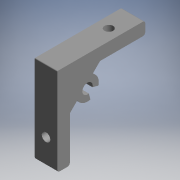
# Autodesk Inventor part: HBLTBS3
Saved by Autodesk Inventor 2017.3 (Build 213256000, 256)
## iProperties
Part Number: HBLTBS3
Material: Generic
Catalog Web Link: www.cadenas.de
Description: HBLTBS3-Square Nuts for Aluminum Extrusions 15mm Square - Extruded Brackets
Vendor: MISUMI
Document SubType Name: Modeling
Designer: partserver
Manufacturer: MISUMI
Mass: 3.67944 g
Surface Area: 22.5843 cm^2
Volume: 3.67944 cm^3
Density: 1 g/cm^3
Appearance: PSOLRGB-175-175-175
Category: PARTsolutions
Company: MISUMI
Title: HBLTBS3
Author: Cadenas PARTsolutions
Comments: Square Nuts for Aluminum Extrusions 15mm Square - Extruded Brackets
PSOL_IDENT_0: {$CADENAS_DATA\23d-libs\misumi\metric\38_al_extrusions_blackets\hbltbs3.prj},155 {VTYP=3D},{NB=HBLTB
PSOL_IDENT_1: S3},{LINA=HBLTBS3},{NN=HBLTBS3},{DATE=08.06.2021 08:27:28},{GEOMDATE=18.09.2018 07:03:18},{VERSION=}
PSOL_IDENT_2: ,{LINEID=10},{WBVAR=},{WBNUMERIC=}  {NB=HBLTBS3},{LINA=HBLTBS3},{KT=DUMMY},{PN=HBLTBS3},{TYPE=HBLTBS
PSOL_IDENT_3: 3},{MAT=6N01SS-T5},{ST=Clear Anodize},{MASS=10},{AE=HFS3-1515},{AS=CBM3-8},{BM=3.000},{BL=8.000},{AS
PSOL_IDENT_4: Q=2},{AN=HNSQ3-3},{ANQ=2},{AL=530}
NB: HBLTBS3
NN: HBLTBS3
NT: Square Nuts for Aluminum Extrusions 15mm Square - Extruded Brackets
NBSYN: $PN.
LINA: HBLTBS3
CATALOG: Misumi
PN: HBLTBS3
TYPE: HBLTBS3
MAT: 6N01SS-T5
ST: Clear Anodize
MASS: 10
AE: HFS3-1515
AS: CBM3-8
ASQ: 2
AN: HNSQ3-3
ANQ: 2
AL: 530
SUPPLIER: MISUMI
ARTICLENO: HBLTBS3
BOMINFO: HBLTBS3
CREATOR: CADENAS GmbH
Autodesk Inventor part; units mm, degrees
ref_plane "YZ Plane" through (0, 0, 0) normal (1, 0, 0) x (0, 1, 0)
ref_plane "XZ Plane" through (0, 0, 0) normal (0, 1, 0) x (-1, 0, 0)
ref_plane "XY Plane" through (0, 0, 0) normal (0, 0, 1) x (1, 0, 0)
sketch "_____1" plane through (0, 0, 0) normal (1, 0, 0) x (0, 0, -1)
  arc A0 (-35, 1) -> (-34, 0) centre (-34, 1) ccw
  line L0 (-34, 0) -> (-0.3, 0)
  arc A1 (-0.3, 0) -> (0, 0.3) centre (-0.3, 0.3) ccw
  line L1 (0, 0.3) -> (0, 34)
  arc A2 (0, 34) -> (-1, 35) centre (-1, 34) ccw
  line L2 (-1, 35) -> (-4, 35)
  arc A3 (-4, 35) -> (-5, 34) centre (-4, 34) ccw
  line L3 (-5, 34) -> (-5, 17.1243)
  arc A4 (-5.0879, 16.9121) -> (-5, 17.1243) centre (-5.3, 17.1243) ccw
  line L4 (-5.0879, 16.9121) -> (-7.6986, 14.3014)
  arc A5 (-8.1663, 14.3564) -> (-7.6986, 14.3014) centre (-7.9107, 14.5135) ccw
  arc A6 (-8.1663, 14.3564) -> (-14.3564, 8.1663) centre (-12, 12) ccw
  arc A7 (-14.3014, 7.6986) -> (-14.3564, 8.1663) centre (-14.5135, 7.9107) ccw
  line L5 (-14.3014, 7.6986) -> (-16.9121, 5.0879)
  arc A8 (-17.1243, 5) -> (-16.9121, 5.0879) centre (-17.1243, 5.3) ccw
  line L6 (-17.1243, 5) -> (-34, 5)
  arc A9 (-34, 5) -> (-35, 4) centre (-34, 4) ccw
  line L7 (-35, 4) -> (-35, 1)
  constraints: 20 point on circle, 16 end point, 10 centre point
extrude "Extrusion1" add sketch "_____1" along normal mid plane 9
sketch "_____2" plane through (0, 0, 0) normal (1, 0, 0) x (0, 0, -1)
  line L0 (-16.8296, 13.2941) -> (-13.9801, 12.5306)
  arc A0 (-13.9801, 12.5306) -> (-12.5306, 13.9801) centre (-12, 12) ccw
  line L1 (-12.5306, 13.9801) -> (-13.2941, 16.8296)
  arc A1 (-13.2941, 16.8296) -> (-16.8296, 13.2941) centre (-12, 12) ccw
  constraints: 4 end point, 4 point on circle, 2 centre point
extrude "Extrusion2" cut sketch "_____2" along normal mid plane 9
sketch "Sketch3" plane through (4.5, 34, 0) normal (0, 0, -1) x (-1, 0, 0)
  point P0 (4.5, -9)
hole "Hole1" at (0, 25, 0) direction (0, 0, 1) diameter 3.4 depth 5
sketch "Sketch4" plane through (-4.5, 5, 34) normal (0, 1, 0) x (1, 0, 0)
  point P0 (4.5, 9)
hole "Hole2" at (0, 5, 25) direction (0, -1, 0) diameter 3.4 depth 5
body "Solid1"
